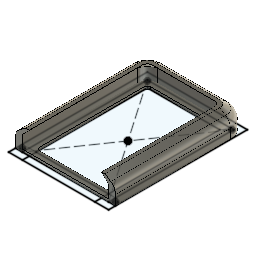
CRYSlight (Autodesk Fusion 360 design; units mm, degrees)
Autodesk Fusion 360 part; units mm, degrees
sketch "clip" plane through (0, 0, 0) normal (0, 0, 1) x (1, 0, 0) in component "clip"
  line L0 (50, 72.5) -> (-50, 72.5)
  line L1 (-50, 72.5) -> (-50, -72.5)
  line L2 (-50, -72.5) -> (50, -72.5)
  line L3 (50, -72.5) -> (50, 72.5)
  line L4 (50, 72.5) -> (-50, -72.5) construction
  line L5 (-50, 72.5) -> (50, -72.5) construction
  line L6 (-42, -64.5) -> (42, -64.5)
  line L7 (42, -64.5) -> (42, 64.5)
  line L8 (42, 64.5) -> (-42, 64.5)
  line L9 (-42, 64.5) -> (-42, -64.5)
  line L10 (-58, 80.5) -> (-58, -80.5)
  line L11 (-58, -80.5) -> (58, -80.5)
  line L12 (58, -80.5) -> (58, 80.5)
  line L13 (58, 80.5) -> (-58, 80.5)
  line L14 (-42, -64.5) -> (-42, -80.5)
  line L15 (42, -64.5) -> (42, -80.5)
  line L16 (50, -72.5) -> (58, -72.5)
  line L17 (-50, -72.5) -> (-58, -72.5)
  line L18 (-42, -64.5) -> (-58, -64.5) construction
  line L19 (42, -64.5) -> (58, -64.5) construction
  line L20 (-50, -72.5) -> (-58, -64.5) construction
  line L21 (-58, -72.5) -> (-50, -64.5) construction
  line L22 (50, -72.5) -> (58, -64.5) construction
  line L23 (58, -72.5) -> (50, -64.5) construction
  circle A0 centre (-54, -68.5) radius 2
  circle A1 centre (54, -68.5) radius 2
  line L24 (42, 64.5) -> (50, 72.5) construction
  circle A2 centre (49.0711, 71.5711) radius 2
  line L25 (-42, 64.5) -> (-50, 72.5) construction
  circle A3 centre (-49.0711, 71.5711) radius 2
  dimension "d1" = 100
  dimension "d2" = 145
  dimension "d5" = -8
  dimension "d12" = 8
  dimension "d44" = 4
  dimension "d45" = 4
  dimension "d49" = 4
  dimension "d50" = 10
  dimension "d53" = 4
  dimension "d54" = 10
  constraint horizontal L0
  constraint perpendicular L0 L1
  constraint parallel L0 L2
  constraint parallel L1 L3
  constraint coincident L4 origin
  constraint coincident L5 origin
  constraint coincident L11 L14.end
  constraint perpendicular L11 L14
  constraint coincident L11 L15.end
  constraint perpendicular L11 L15
  constraint coincident L12 L16.end
  constraint perpendicular L12 L16
  constraint coincident L10 L17.end
  constraint perpendicular L10 L17
  constraint coincident L10 L18.end
  constraint perpendicular L10 L18
  constraint coincident L12 L19.end
  constraint perpendicular L12 L19
  constraint midpoint L18 L21.end
  constraint midpoint L19 L23.end
  constraint midpoint L21 A0.centre
  constraint midpoint L23 A1.centre
  constraint coincident L24 A2.centre
  constraint coincident L25 A3.centre
  measures "d1" distance of L1.end L2.end
  measures "d2" distance of L0.end L1.end
  measures "d44" diameter of A0
  measures "d45" diameter of A1
  measures "d49" diameter of A2
  measures "d50" distance of L7.end A2.centre
  measures "d53" diameter of A3
  measures "d54" distance of L8.end A3.centre
extrude "Extrude1" add sketch "clip" along normal blind 26 contours L0 L3 A2 | L0 L3 A2 | L0 L1 L2 L3 L7 L8 L9 L14 L15 A2 A3 | L0 L1 L3 L10 L12 L13 L16 L17 A2 A3 | L0 L1 A3 | L0 L1 A3 | L2 L6 L14 L15 | L6 L7 L8 L9 | A0 | A1 in component "clip"
extrude "Extrude3" cut sketch "clip" along normal blind 26 contours L6 L7 L8 L9 in component "clip"
extrude "Extrude4" cut sketch "clip" along normal blind 15 from surface at 3 contours L0 L3 A2 | L0 L1 L2 L3 L7 L8 L9 L14 L15 A2 A3 | L0 L1 A3 | L2 L6 L14 L15 picked at (48.4405, 70.9405) picked at (-48.4608, 70.9205) in component "clip"
extrude "Extrude7" cut sketch "clip" along normal blind 23 from surface at 3 contours L2 L6 L14 L15 in component "clip"
fillet "Fillet2" radius 12 2 edges at (50, 72.5, 10.5) (-50, 72.5, 10.5) in component "clip"
fillet "Fillet2" radius 6 2 edges at (42, 64.5, 22) (-42, 64.5, 22) in component "clip"
fillet "Fillet2" radius 20 2 edges at (58, 80.5, 13) (-58, 80.5, 13) in component "clip"
fillet "Fillet2" radius 4 4 edges at (42, 64.5, 1.5) (-42, 64.5, 1.5) (-42, -64.5, 1.5) (42, -64.5, 1.5) in component "clip"
extrude "Extrude8" cut sketch "clip" along normal blind 10 contours L0 L3 A2 | L0 L3 A2 | L0 L1 A3 | L0 L1 A3 | A0 | A1 in component "clip"
chamfer "Chamfer2" distance 7.95 angle 45 5 edges at (-42, -7, 18) (-40.2426, 62.7426, 18) (0, 64.5, 18) (40.2426, 62.7426, 18) (42, -7, 18) in component "clip"
chamfer "Chamfer2" distance 12 distance2 8 5 edges at (58, -6, 26) (52.1421, 74.6421, 26) (0, 80.5, 26) (-52.1421, 74.6421, 26) (-58, -6, 26) measured on face at (-52.6667, 15.5, 26) measured on face at (38.9516, 80.4773, 8.6667) measured on face at (-52.6667, 15.5, 26) measured on face at (-38.9516, 80.4773, 8.6667) measured on face at (-52.6667, 15.5, 26) in component "clip"
fillet "Fillet3" radius 12 5 edges at (58, -6, 18) (52.1421, 74.6421, 18) (0, 80.5, 18) (-52.1421, 74.6421, 18) (-58, -6, 18) in component "clip"
component "clip" placed x (1, 0, 0) y (0, 1, 0) z (0, 0, 1) at (0, 0, 0)
component "shader" placed x (1, 0, 0) y (0, 1, 0) z (0, 0, 1) at (0, 0, 0)
named bodies: "clipBody"
